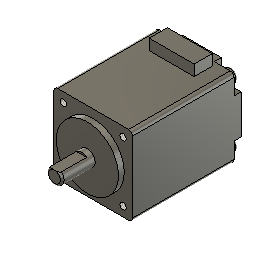
NEMA8 Stepper Motor v2 (Autodesk Fusion 360 design; units mm, degrees)
Autodesk Fusion 360 part; units mm, degrees
sketch "Sketch2" plane through (0, 0, 0) normal (0, 0, 1) x (1, 0, 0)
  line L0 (-9.15, 10.15) -> (9.15, 10.15)
  line L1 (10.15, 9.15) -> (10.15, -9.15)
  line L2 (9.15, -10.15) -> (-9.15, -10.15)
  line L3 (-10.15, -9.15) -> (-10.15, 9.15)
  line L4 (0, 10.15) -> (0, -10.15) construction
  line L5 (-10.15, 0) -> (10.15, 0) construction
  circle A0 centre (0, 0) radius 8
  circle A1 centre (0, 0) radius 2
  circle A2 centre (7.7, 7.7) radius 1
  circle A3 centre (-7.7, 7.7) radius 1
  circle A4 centre (-7.7, -7.7) radius 1
  circle A5 centre (7.7, -7.7) radius 1
  line L6 (-7.7, 7.7) -> (7.7, 7.7) construction
  line L7 (7.7, 7.7) -> (7.7, -7.7) construction
  line L8 (7.7, -7.7) -> (-7.7, -7.7) construction
  line L9 (-7.7, -7.7) -> (-7.7, 7.7) construction
  line L10 (-1.3229, 1.5) -> (1.3229, 1.5)
  arc A6 (-9.15, 10.15) -> (-10.15, 9.15) centre (-9.15, 9.15) ccw
  arc A7 (10.15, 9.15) -> (9.15, 10.15) centre (9.15, 9.15) ccw
  arc A8 (-10.15, -9.15) -> (-9.15, -10.15) centre (-9.15, -9.15) ccw
  arc A9 (9.15, -10.15) -> (10.15, -9.15) centre (9.15, -9.15) ccw
  dimension "d2" = 20.3
  dimension "d3" = 15.4
  dimension "d4" = 2
  dimension "d5" = 7.7
  dimension "d6" = 7.7
  dimension "d7" = 16
  dimension "d8" = 4
  dimension "d9" = 3.5
  dimension "d10" = 1
  constraint horizontal L0
  constraint vertical L1
  constraint horizontal L2
  constraint vertical L3
  constraint coincident A0.centre L5
  constraint coincident A0.centre L4
  constraint coincident A0.centre A1.centre
  constraint horizontal L6
  constraint vertical L7
  constraint horizontal L8
  constraint vertical L9
  constraint equal L6 L7
  constraint equal A3 A4
  constraint equal A4 A5
  constraint equal A2 A5
  constraint coincident A4.centre L8.end
  constraint coincident A3.centre L6.start
  constraint coincident A2.centre L6.end
  constraint coincident A5.centre L7.end
  constraint coincident A1 L10.start
  constraint coincident A1 L10.end
  constraint perpendicular L4 L10
  constraint coincident L0 L4.start
  constraint coincident L3 L5.start
  constraint tangent L0 A6
  constraint tangent L3 A6
  constraint coincident L1 L5.end
  constraint tangent L0 A7
  constraint tangent L1 A7
  constraint equal A6 A7
  constraint coincident L2 L4.end
  constraint tangent L2 A8
  constraint tangent L3 A8
  constraint equal A6 A8
  constraint tangent L1 A9
  constraint tangent L2 A9
  constraint equal A6 A9
  measures "d2" distance of L1 L3
  measures "d3" distance of L6 L8
  measures "d4" diameter of A4
  measures "d5" distance of A0.centre L8
  measures "d6" distance of L4 L7
  measures "d7" diameter of A0
  measures "d8" diameter of A1
  measures "d10" radius of A6
extrude "Extrude1" add sketch "Sketch2" against normal blind 28 contours L0 L1 L2 L3 A6 A7 A8 A9 | A0 | A1 L10 | A1 L10 | A2 | A3 | A4 | A5 makes body 1
extrude "Extrude2" add sketch "Sketch2" along normal blind 1.5 contours A0 | A1 L10 | A1 L10 bodies 1
extrude "Extrude3" add sketch "Sketch2" along normal blind 10 contours A1 L10 picked at (0.3407, 0.427) bodies 1
extrude "Extrude4" add sketch "Sketch2" along normal blind 3 contours A1 L10 picked at (0.096, 1.6597) bodies 1
fillet "Fillet1" radius 0.5 1 edges at (0, -2, 10) on bodies 1
hole "Hole1" at (-7.7, 7.7, 0) at (7.7, 7.7, 0) at (7.7, -7.7, 0) at (-7.7, -7.7, 0) direction (0, 0, -1) diameter 1.623 depth 2.5 tip angle 118 bodies 1
thread "Thread1" "ISO Metric profile 2.0 M2x0.4 6H"
sketch "Sketch3" plane through (0, 10.15, 0) normal (0, 1, 0) x (-1, 0, 0)
  line L0 (9.15, 0) -> (-9.15, 0)
  line L1 (-9.15, 0) -> (-9.15, -28)
  line L2 (-9.15, -28) -> (9.15, -28)
  line L3 (9.15, -28) -> (9.15, 0)
  line L4 (5.8, -24.925) -> (-5.8, -24.925)
  line L5 (-5.8, -24.925) -> (-5.8, -20.25)
  line L6 (-5.8, -20.25) -> (5.8, -20.25)
  line L7 (5.8, -20.25) -> (5.8, -24.925)
  line L8 (0, -24.925) -> (0, -20.25) construction
  point P0 (0, -28)
  dimension "d23" = 11.6
  dimension "d24" = 4.675
  dimension "d25" = 3.075
  constraint horizontal L4
  constraint vertical L5
  constraint horizontal L6
  constraint vertical L7
  constraint midpoint L4 L8.start
  constraint midpoint L6 L8.end
  constraint midpoint L2 P0
  constraint coincident L8 P0
  measures "d23" distance of L4.start L4.end
  measures "d24" distance of L4.end L5.end
  measures "d25" distance of L2 L4
extrude "Extrude5" add sketch "Sketch3" along normal blind 2.8 contours L4 L5 L6 L7 bodies 1
sketch "Sketch4" plane through (0, 0, -28) normal (0, 0, -1) x (-1, 0, 0)
  arc A0 (9.15, -10.15) -> (10.15, -9.15) centre (9.15, -9.15) ccw
  line L0 (10.15, -9.15) -> (10.15, 9.15)
  arc A1 (10.15, 9.15) -> (9.15, 10.15) centre (9.15, 9.15) ccw
  line L1 (9.15, 10.15) -> (-9.15, 10.15)
  arc A2 (-9.15, 10.15) -> (-10.15, 9.15) centre (-9.15, 9.15) ccw
  line L2 (-10.15, 9.15) -> (-10.15, -9.15)
  arc A3 (-10.15, -9.15) -> (-9.15, -10.15) centre (-9.15, -9.15) ccw
  line L3 (-9.15, -10.15) -> (9.15, -10.15)
  circle A4 centre (0, 0) radius 2.75
  circle A5 centre (7.7, 7.7) radius 0.8115
  circle A6 centre (-7.7, 7.7) radius 0.8115
  circle A7 centre (-7.7, -7.7) radius 0.8115
  circle A8 centre (7.7, -7.7) radius 0.8115
  circle A9 centre (-7.7, 7.7) radius 1.65
  circle A10 centre (7.7, 7.7) radius 1.65
  circle A11 centre (7.7, -7.7) radius 1.65
  circle A12 centre (-7.7, -7.7) radius 1.65
  line L4 (-5.05, 10.15) -> (-5.05, 7.05)
  line L5 (-7.05, 5.05) -> (-10.15, 5.05)
  line L6 (5.05, 10.15) -> (5.05, 7.05)
  line L7 (7.05, 5.05) -> (10.15, 5.05)
  line L8 (10.15, -5.05) -> (7.05, -5.05)
  line L9 (5.05, -7.05) -> (5.05, -10.15)
  line L10 (-5.05, -10.15) -> (-5.05, -7.05)
  line L11 (-7.05, -5.05) -> (-10.15, -5.05)
  arc A13 (-7.05, 5.05) -> (-5.05, 7.05) centre (-7.05, 7.05) ccw
  arc A14 (5.05, 7.05) -> (7.05, 5.05) centre (7.05, 7.05) ccw
  arc A15 (7.05, -5.05) -> (5.05, -7.05) centre (7.05, -7.05) ccw
  arc A16 (-5.05, -7.05) -> (-7.05, -5.05) centre (-7.05, -7.05) ccw
  point P0 (5.05, 5.05)
  dimension "d28" = 3.3
  dimension "d29" = 5.1
  dimension "d30" = 2
  dimension "d34" = 5.5
  constraint coincident A4.centre origin
  constraint concentric A6 A9
  constraint concentric A5 A10
  constraint concentric A8 A11
  constraint concentric A7 A12
  constraint equal A9 A12
  constraint equal A9 A10
  constraint equal A10 A11
  constraint coincident L1 L4.start
  constraint perpendicular L1 L4
  constraint coincident L2 L5.end
  constraint perpendicular L2 L5
  constraint coincident L1 L6.start
  constraint perpendicular L1 L6
  constraint coincident L0 L7.end
  constraint perpendicular L0 L7
  constraint coincident L0 L8.start
  constraint perpendicular L0 L8
  constraint coincident L3 L9.end
  constraint perpendicular L3 L9
  constraint coincident L3 L10.start
  constraint perpendicular L3 L10
  constraint coincident L2 L11.end
  constraint perpendicular L2 L11
  constraint collinear L4 L10
  constraint collinear L5 L7
  constraint collinear L6 L9
  constraint collinear L8 L11
  constraint tangent L5 A13
  constraint tangent L4 A13
  constraint coincident P0 L6
  constraint coincident P0 L7
  constraint tangent L6 A14
  constraint tangent L7 A14
  constraint equal A13 A14
  constraint tangent L8 A15
  constraint tangent L9 A15
  constraint equal A13 A15
  constraint tangent L10 A16
  constraint tangent L11 A16
  constraint equal A13 A16
  measures "d28" diameter of A12
  measures "d29" distance of P0 L7.end
  measures "d30" radius of A13
  measures "d34" diameter of A4
extrude "Extrude6" cut sketch "Sketch4" against normal blind 1.8 contours A0 L0 L3 L8 L9 A15 | L2 A3 L3 L10 L11 A16 | L0 A1 L1 L6 L7 A14 | L1 A2 L2 L4 L5 A13 bodies 1
fillet "Fillet2" radius 0.5 4 edges at (9.2383, 7.1033, -28) (9.2383, -8.2967, -28) (-6.1617, 7.1033, -28) (-6.1617, -8.2967, -28) on bodies 1
extrude "Extrude7" cut sketch "Sketch4" against normal blind 4.3 contours A4 bodies 1
split "Split1" by plane through (0, 0, 1.5) normal (0, 0, 1) bodies 1 makes body 2 at (-1.487, 1.3374, 4.6667)
copy_body "Body->Comp1" bodies 2 removing the originals makes body 3 in component "Shaft"
component "Shaft" placed x (1, 0, 0) y (0, 1, 0) z (0, 0, 1) at (0, 0, 0)
equation "d5 = d3 / 2"
equation "d6 = d5"
